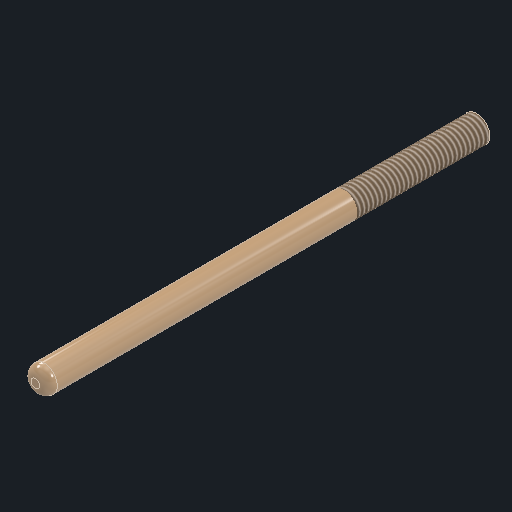
# Autodesk Inventor part: Domed End Rod 40mm
Saved by Autodesk Inventor 2027.1 (Build 311270010, 270A)
## iProperties
Created: 2025-09-16
Part Number: Domed End Rod 40mm
Material: Stainless Steel
Document SubType Name: Modeling
Designer: SD
Density: 8 g/cm^3
Appearance: Brindle
Mass: 2.49379 g
Surface Area: 3.86638 cm^2
Volume: 0.281022 cm^3
Project: Automatic Tea Steeping mechanism
Length: 50.000 mm
BOM-Mass: 0.00249
BOM-Area: 0.000
Diameter: 3.000 mm
Procurement: Fabricate - 1st round
Build Stage: 1
Preferred Material: 303 Stainless Steel
Author: SD
Title: Domed End Rod 40mm
Autodesk Inventor part; units mm, degrees
ref_plane "YZ Plane" through (0, 0, 0) normal (1, 0, 0) x (0, 1, 0)
ref_plane "XZ Plane" through (0, 0, 0) normal (0, 1, 0) x (-1, 0, 0)
ref_plane "XY Plane" through (0, 0, 0) normal (0, 0, 1) x (1, 0, 0)
sketch "Sketch1" plane through (0, 0, 0) normal (0, 0, 1) x (1, 0, 0)
  circle A0 centre (0, 0) radius 1.5
  dimension "Diameter" = 3
  constraints: 1 centre point, 1 coincident
  measures "Diameter" diameter of A0
extrude "Extrusion1" add sketch "Sketch1" along normal mid plane 50
thread "Thread1" size "M3x0.5" class "6g" standard "ISO Metric profile" length 15
fillet "Fillet1" radius 1 1 edges at (-1.5, 0, 25)
body "Solid1"
